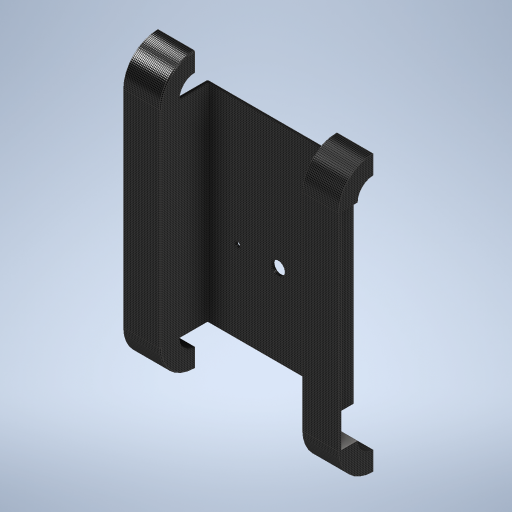
# Autodesk Inventor part: body base
Saved by Autodesk Inventor 2024 (Build 280153000, 153)
## iProperties
Created: 2023-06-28
Part Number: body base
Material: Steel, Alloy
Document SubType Name: Modeling
Designer: Anshul
Density: 7.73 g/cm^3
Appearance: Semi-Polished
Author: Anshul
Autodesk Inventor part; units mm, degrees
ref_plane "XY Plane" through (0, 0, 0) normal (0, 0, 1) x (1, 0, 0)
sketch "Sketch1" plane through (0, 0, 0) normal (0, 0, 1) x (1, 0, 0)
  line L0 (0, 0) -> (270, 0)
  line L1 (270, 0) -> (270, 380)
  line L2 (270, 380) -> (0, 380)
  line L3 (0, 380) -> (0, 0)
  dimension "d0" = 270
  dimension "d1" = 380
  constraints: 8 end point, 2 parallel, 1 horizontal, 1 perpendicular
  measures "d0" distance of L2.end L1.end
  measures "d1" distance of L1.end L0.end
extrude "Extrusion1" add sketch "Sketch1" along normal blind 5
sketch "Sketch4" plane through (0, 0, 0) normal (-1, 0, 0) x (0, 0, 1)
  line L0 (0, 0) -> (0, 380) projected
  line L1 (-3.8919, 9.8795) -> (0, 9.8795)
  line L2 (0, 9.8795) -> (0, 5.6882)
  line L3 (0, 5.6882) -> (-3.8919, 5.6882)
  line L4 (-3.8919, 5.6882) -> (-3.8919, 9.8795)
  line L5 (5, 0) -> (5, 380) projected
  line L6 (5, 380) -> (87, 380)
  line L7 (87, 380) -> (87, 0)
  line L8 (87, 0) -> (5, 0)
  line L9 (5, 0) -> (5, 380)
  dimension "d4" = 82
  dimension "d5" = 380
  constraints: 16 end point, 4 parallel, 2 horizontal, 2 perpendicular, 1 point on line
  measures "d4" distance of L7.end L8.end
  measures "d5" distance of L6.end L7.end
extrude "Extrusion2" add sketch "Sketch4" against normal blind 5 contours L5 L6 L7 L8
sketch "Sketch7" plane through (0, 0, 0) normal (-1, 0, 0) x (0, 0, 1)
  line L0 (0, 380) -> (87, 380) projected
  line L1 (87, 380) -> (92, 380)
  line L2 (92, 380) -> (92, 0)
  line L3 (92, 0) -> (87, 0)
  line L4 (87, 0) -> (87, 380)
  point P0 (0, 0)
  dimension "d8" = 5
  dimension "d9" = 380
  constraints: 8 end point, 2 parallel, 1 horizontal, 1 perpendicular
  measures "d8" distance of L2.end L3.end
  measures "d9" distance of L1.end L2.end
extrude "Extrusion3" add sketch "Sketch7" along normal blind 63 and the other way blind 5
sketch "Sketch8" plane through (0, 0, 0) normal (-1, 0, 0) x (0, 0, 1)
  line L0 (0, 380) -> (5, 380) projected
  line L1 (0, 380) -> (0, 390)
  line L2 (0, 390) -> (1.5922, 390)
  line L3 (5, 380) -> (92, 380) projected
  arc A0 (92, 380) -> (28.5, 443.5) centre (28.5, 380) ccw
  line L4 (28.5, 408.706) -> (28.5, 443.5)
  line L5 (57.206, 380) -> (92, 380)
  arc A1 (57.206, 380) -> (28.5, 408.706) centre (28.5, 380) ccw
  arc A2 (1.5922, 390) -> (0, 383.4325) centre (28.5, 380) ccw
  point P0 (0, 0)
  dimension "d14" = 10
  constraints: 8 end point, 7 point on circle, 3 centre point, 2 point on line, 2 vertical, 1 coincident
  measures "d14" distance of L0.start L1.end
extrude "Extrusion4" add sketch "Sketch8" along normal blind 63 and the other way blind 5 contours A1 L4 A0 L3
ref_plane "Work Plane1" through (0, 190, 0) normal (0, 1, 0) x (-1, 0, 0)
mirror "Mirror1" about plane through (0, 190, 0) normal (0, 1, 0) of "Extrusion4"
ref_plane "Work Plane3" through (135, 0, 0) normal (1, 0, 0) x (0, 1, 0)
mirror "Mirror2" about plane through (135, 0, 0) normal (1, 0, 0) of "Extrusion4", "Extrusion3", "Mirror1", "Extrusion2"
fillet "Fillet1" radius 2 3 edges at (5, -44.9013, 73.4013) (5, 424.9013, 73.4013) (5, 190, 92)
fillet "Fillet2" radius 2 3 edges at (265, 190, 92) (265, -44.9013, 73.4013) (265, 424.9013, 73.4013)
fillet "Fillet3" radius 2 1 edges at (5, 190, 5)
fillet "Fillet4" radius 2 1 edges at (265, 190, 5)
fillet "Fillet5" radius 2 1 edges at (0, 190, 0)
fillet "Fillet6" radius 2 1 edges at (270, 190, 0)
sketch "Sketch9" plane through (0, 0, 5) normal (0, 0, 1) x (1, 0, 0)
  line L0 (7, 0) -> (263, 0) construction
  line L1 (135, 0) -> (135, 150) construction
  circle A0 centre (135, 150) radius 12.5
  line L2 (135, 150) -> (258, 150) construction
  line L3 (135, 150) -> (12, 150) construction
  circle A1 centre (210, 150) radius 5
  circle A2 centre (60, 150) radius 5
  line L4 (5, 0) -> (5, 380) projected
  line L5 (265, 380) -> (265, 0) projected
  point P0 (0, 0)
  dimension "d27" = 150
  dimension "d28" = 25
  dimension "d31" = 10
  dimension "d32" = 10
  dimension "d33" = 55
  dimension "d34" = 55
  constraints: 6 end point, 3 centre point, 2 horizontal, 2 point on line, 1 coincident, 1 midpoint, 1 vertical
  measures "d27" distance of L1.start L1.end
  measures "d28" diameter of A0
  measures "d31" diameter of A1
  measures "d32" diameter of A2
  measures "d33" distance from line of A2.centre L4
  measures "d34" distance from line of A1.centre L5
extrude "Extrusion5" cut sketch "Sketch9" against normal through all
body "Solid1"
